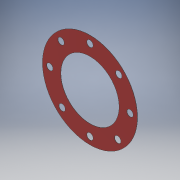
# Autodesk Inventor part: reverse gear up cylinder packing
Saved by Autodesk Inventor 2017 (Build 210142000, 142)
## iProperties
Created: 2018-11-07
Part Number: reverse gear up cylinder packing
Material: Generic
Document SubType Name: Modeling
Designer: User
Density: 1 g/cm^3
Appearance: Default
Author: User
Autodesk Inventor part; units mm, degrees
ref_plane "YZ Plane" through (0, 0, 0) normal (1, 0, 0) x (0, 1, 0)
ref_plane "XZ Plane" through (0, 0, 0) normal (0, 1, 0) x (-1, 0, 0)
ref_plane "XY Plane" through (0, 0, 0) normal (0, 0, 1) x (1, 0, 0)
sketch "Sketch1" plane through (0, 0, 0) normal (0, 1, 0) x (-1, 0, 0)
  circle A0 centre (0, 0) radius 26
  circle A1 centre (0, 0) radius 16
  circle A2 centre (0, 0) radius 22 construction
  circle A3 centre (0, 22) radius 1.75
  circle A4 centre (0, -22) radius 1.75
  circle A5 centre (22, 0) radius 1.75
  circle A6 centre (-22, 0) radius 1.75
  circle A7 centre (15.2274, -15.8785) radius 1.75
  circle A8 centre (-15.8099, 15.2986) radius 1.75
  circle A9 centre (15.8099, 15.2986) radius 1.75
  circle A10 centre (-15.2274, -15.8785) radius 1.75
  dimension "d2" = 44
  dimension "d0" = 52
  dimension "d1" = 32
  dimension "d21" = 3.5
  dimension "d22" = 3.5
  dimension "d23" = 3.5
  dimension "d24" = 3.5
  dimension "d25" = 3.5
  dimension "d26" = 3.5
  dimension "d27" = 3.5
  dimension "d28" = 3.5
  constraints: 10 centre point, 3 coincident, 10 other
  measures "d0" diameter of A0
  measures "d1" diameter of A1
  measures "d21" diameter of A3
  measures "d22" diameter of A4
  measures "d23" diameter of A5
  measures "d24" diameter of A6
  measures "d25" diameter of A7
  measures "d26" diameter of A8
  measures "d27" diameter of A9
  measures "d28" diameter of A10
extrude "Extrusion2" add sketch "Sketch1" along normal blind 0.1
body "Solid2"
